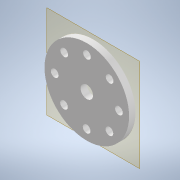
# Autodesk Inventor part: servo flange
Saved by Autodesk Inventor 2021 (Build 250183000, 183)
## iProperties
Created: 2021-11-20
Part Number: servo flange
Material: Generic
Document SubType Name: Modeling
Designer: techv
Density: 1 g/cm^3
Appearance: Default
Author: techv
Autodesk Inventor part; units mm, degrees
ref_plane "YZ Plane" through (0, 0, 0) normal (1, 0, 0) x (0, 1, 0)
ref_plane "XZ Plane" through (0, 0, 0) normal (0, 1, 0) x (-1, 0, 0)
ref_plane "XY Plane" through (0, 0, 0) normal (0, 0, 1) x (1, 0, 0)
ref_plane "Work Plane1" through (0, 0, 0) normal (0, 0, 1) x (1, 0, 0)
sketch "Sketch1" plane through (0, 0, 0) normal (0, 0, 1) x (1, 0, 0)
  circle A0 centre (0, 0) radius 19.75 projected
  circle A1 centre (-14.9998, 0.0716) radius 1.8 projected
  circle A2 centre (0, 0) radius 5.5 projected
  circle A3 centre (-10.6571, -10.5558) radius 1.8 projected
  circle A4 centre (-0.0716, -14.9998) radius 1.8 projected
  circle A5 centre (10.5558, -10.6571) radius 1.8 projected
  circle A6 centre (14.9998, -0.0716) radius 1.8 projected
  circle A7 centre (10.6571, 10.5558) radius 1.8 projected
  circle A8 centre (0.0716, 14.9998) radius 1.8 projected
  circle A9 centre (-10.5558, 10.6571) radius 1.8 projected
  circle A10 centre (0, 0) radius 2.92
  point P0 (0, 0)
  point P1 (1.2639, -2.6323)
  constraints: 1 coincident, 4 other
extrude "Extrusion1" add sketch "Sketch1" along normal blind 3 contours A0 | A2
body "Solid1"
